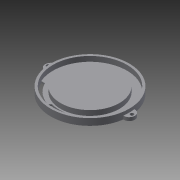
# Autodesk Inventor part: clock_case
Saved by Autodesk Inventor 2015 SP2 (Build 190223200, 223)
## iProperties
Created: 2016-02-29
Part Number: clock_case
Material: Generic
Document SubType Name: Modeling
Designer: mca20
Density: 1 g/cm^3
Appearance: Default
Author: mca20
Autodesk Inventor part; units mm, degrees
ref_plane "YZ Plane" through (0, 0, 0) normal (1, 0, 0) x (0, 1, 0)
ref_plane "XZ Plane" through (0, 0, 0) normal (0, 1, 0) x (-1, 0, 0)
ref_plane "XY Plane" through (0, 0, 0) normal (0, 0, 1) x (1, 0, 0)
sketch "Sketch1" plane through (0, 0, 0) normal (0, 1, 0) x (-1, 0, 0)
  circle A0 centre (0, 0) radius 26.25
  circle A1 centre (0, 0) radius 33
  dimension "d0" = 52.5
  dimension "d1" = 66
  constraints: 2 centre point, 2 coincident
  measures "d0" diameter of A0
  measures "d1" diameter of A1
extrude "Extrusion1" add sketch "Sketch1" along normal blind 1.5
sketch "Sketch2" plane through (0, 1.5, 0) normal (0, 1, 0) x (1, 0, 0)
  circle A0 centre (0, 0) radius 27.5
  circle A1 centre (0, 0) radius 33 projected
  line L0 (-7.5, -26.4575) -> (-11.8438, -30.8014)
  circle A2 centre (0, 0) radius 33 projected
  line L1 (-7.5, -26.4575) -> (-1.3569, -26.4575) construction
  line L2 (7.5, -26.4575) -> (11.8438, -30.8014)
  line L3 (7.5, -26.4575) -> (13.6431, -26.4575) construction
  point P0 (0, -27.5)
  dimension "d4" = 55
  dimension "d5" = 135
  dimension "d6" = 45
  dimension "d7" = 15
  dimension "d9" = 7.5
  dimension "d10" = 0
  constraints: 8 end point, 5 point on circle, 2 equal length, 2 horizontal, 1 centre point, 1 coincident
  measures "d4" diameter of A0
  measures "d5" angle of L0 L1
  measures "d6" angle of L2 L3
  measures "d7" distance of L2.start L0.start
  measures "d9" horizontal distance of point (0, -27.5) L2.start
  measures "d10" horizontal distance of point (0, -27.5) A0.centre
extrude "Extrusion2" cut sketch "Sketch2" against normal blind 1.5 contours A0 L2 A1 L0 picked at (0.8428, -30.9633)
sketch "Sketch3" plane through (0, 1.5, 0) normal (0, 1, 0) x (1, 0, 0)
  circle A0 centre (0, 0) radius 30
  arc A1 (11.8438, -30.8014) -> (-11.8438, -30.8014) centre (0, 0) ccw projected
  line L0 (7.5, -26.4575) -> (11.8438, -30.8014) projected
  line L1 (-26.8544, -13.3731) -> (-30.1689, -13.3731)
  arc A2 (11.8438, -30.8014) -> (-11.8438, -30.8014) centre (0, 0) ccw projected
  line L2 (-26.8544, -13.3731) -> (-23.54, -13.3731) construction
  line L3 (26.8544, -13.3731) -> (30.1758, -13.3574)
  line L4 (-9.6719, -28.6294) -> (-11.8438, -30.8014)
  line L5 (11.8438, -30.8014) -> (7.5, -26.4575) projected
  line L6 (9.4989, -28.4565) -> (11.8438, -30.8014)
  line L7 (-7.5, -26.4575) -> (-11.8438, -30.8014) projected
  line L8 (-9.4989, -28.4565) -> (-11.8438, -30.8014)
  dimension "d13" = 60
  dimension "d14" = 180
  constraints: 12 end point, 7 point on circle, 3 collinear, 2 point on line, 1 centre point, 1 coincident, 1 horizontal
  measures "d13" diameter of A0
  measures "d14" angle of L1 L2
extrude "Extrusion3" cut sketch "Sketch3" against normal blind 10 contours A0 L7 L4 A1 L1 | L3 A1 L0 A0
sketch "Sketch4" plane through (0, 1.5, 0) normal (0, 1, 0) x (1, 0, 0)
  circle A0 centre (0, 0) radius 26.25 projected
  circle A1 centre (0, 0) radius 22.5
  dimension "d22" = 45
  dimension "d23" = 52.5
  constraints: 1 centre point, 1 coincident
  measures "d22" diameter of A1
  measures "d23" diameter of A0
extrude "Extrusion4" add sketch "Sketch4" against normal blind 1.5 contours A0 | A1
sketch "Sketch5" plane through (0, 0, 0) normal (0, -1, 0) x (1, 0, 0)
  circle A0 centre (0, 0) radius 22.5
  dimension "d19" = 45
  constraints: 1 centre point, 1 coincident
  measures "d19" diameter of A0
extrude "Extrusion5" cut sketch "Sketch5" against normal blind 5
sketch "Sketch6" plane through (0, 1.5, 0) normal (0, 1, 0) x (1, 0, 0)
  circle A0 centre (0, 0) radius 26.25
  circle A1 centre (0, 0) radius 22.5 projected
  dimension "d24" = 52.5
  constraints: 1 centre point, 1 coincident
  measures "d24" diameter of A0
extrude "Extrusion6" add sketch "Sketch6" along normal blind 3.5
sketch "Sketch7" plane through (0, 5, 0) normal (0, 1, 0) x (1, 0, 0)
  circle A0 centre (0, 0) radius 26.25 projected
extrude "Extrusion7" add sketch "Sketch7" along normal blind 1
sketch "Sketch8" plane through (0, 0, 0) normal (0, -1, 0) x (1, 0, 0)
  circle A0 centre (0, 0) radius 33
  circle A1 centre (0, 0) radius 35
  dimension "d29" = 66
  dimension "d30" = 2
  constraints: 2 centre point, 1 coincident
  measures "d29" diameter of A0
  measures "d30" radial gap between concentric circles of A0 A1
extrude "Extrusion8" add sketch "Sketch8" against normal blind 6
sketch "Sketch9" plane through (0, 0, 0) normal (0, -1, 0) x (1, 0, 0)
  circle A0 centre (0, 0) radius 35 projected
  circle A1 centre (-35, 0) radius 5
  circle A2 centre (35, 0) radius 5
  circle A3 centre (0, 0) radius 35 projected
  point P0 (34.6429, 4.9872)
  point P1 (34.6429, -4.9872)
  point P2 (-34.6429, -4.9872)
  point P3 (-34.6429, 4.9872)
  point P4 (-34.6429, -4.9872)
  point P5 (-34.6429, 4.9872)
  dimension "d33" = 10
  dimension "d34" = 10
  constraints: 9 point on circle, 4 coincident, 2 centre point
  measures "d33" diameter of A1
  measures "d34" diameter of A2
extrude "Extrusion9" add sketch "Sketch9" against normal blind 3 contours A0 A2 picked at (36.4733, -1.3095)
sketch "Sketch10" plane through (0, 0, 0) normal (0, -1, 0) x (1, 0, 0)
  arc A0 (34.6429, 4.9872) -> (34.6429, -4.9872) centre (0, 0) ccw projected
  circle A1 centre (-35, 0) radius 5
  circle A2 centre (0, 0) radius 35 projected
  point P0 (-34.6429, -4.9872)
  point P1 (-34.6429, 4.9872)
  dimension "d37" = 10
  constraints: 5 point on circle, 1 centre point
  measures "d37" diameter of A1
extrude "Extrusion10" add sketch "Sketch10" against normal blind 3 contours A0 A1 picked at (-36.6402, 0)
sketch "Sketch11" plane through (0, 3, 0) normal (0, 1, 0) x (1, 0, 0)
  arc A0 (34.6429, -4.9872) -> (34.6429, 4.9872) centre (35, 0) ccw projected
  circle A1 centre (37.5, 0) radius 1.5
  point P0 (0, 0)
  dimension "d40" = 2.5
  dimension "d41" = 3
  constraints: 1 centre point, 1 coincident
  measures "d40" distance of A0.centre point (37.5, 0)
  measures "d41" diameter of A1
hole "Hole1" at (37.5, 3, 0) direction (0, -1, 0) diameter 3 end through all
sketch "Sketch13" plane through (0, 3, 0) normal (0, 1, 0) x (1, 0, 0)
  arc A0 (-34.6429, 4.9872) -> (-34.6429, -4.9872) centre (-35, 0) ccw projected
  circle A1 centre (-37.5, 0) radius 1.5
  point P0 (0, 0)
  dimension "d49" = 2.5
  dimension "d50" = 3
  constraints: 1 centre point, 1 coincident
  measures "d49" distance of A0.centre point (-37.5, 0)
  measures "d50" diameter of A1
hole "Hole2" at (-37.5, 3, 0) direction (0, -1, 0) diameter 3 end through all
sketch "Sketch14" plane through (0, 0, 0) normal (0, -1, 0) x (1, 0, 0)
  circle A0 centre (0, 0) radius 25
  dimension "d58" = 50
  constraints: 1 centre point, 1 coincident
  measures "d58" diameter of A0
extrude "Extrusion11" cut sketch "Sketch14" against normal blind 2
body "Solid1"
